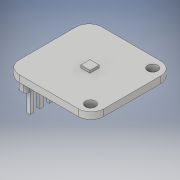
# Autodesk Inventor part: Adafruit TMP007 IR Sensor
Saved by Autodesk Inventor 2018 (Build 220112000, 112)
## iProperties
Created: 2018-10-23
Part Number: Adafruit TMP007 IR Sensor
Material: Generic
Document SubType Name: Modeling
Designer: tbrow
Density: 1 g/cm^3
Appearance: Default
Author: tbrow
Autodesk Inventor part; units mm, degrees
ref_plane "YZ Plane" through (0, 0, 0) normal (1, 0, 0) x (0, 1, 0)
ref_plane "XZ Plane" through (0, 0, 0) normal (0, 1, 0) x (-1, 0, 0)
ref_plane "XY Plane" through (0, 0, 0) normal (0, 0, 1) x (1, 0, 0)
sketch "Sketch1" plane through (0, 0, 0) normal (0, 1, 0) x (-1, 0, 0)
  line L0 (3.175, 0) -> (17.653, 0)
  line L1 (20.828, -3.175) -> (20.828, -17.145)
  line L2 (17.653, -20.32) -> (3.175, -20.32)
  line L3 (0, -17.145) -> (0, -3.175)
  circle A0 centre (2.6416, -2.5146) radius 1.2446
  circle A1 centre (2.6416, -17.8054) radius 1.2446
  line L4 (1.397, -2.5146) -> (0, -2.5146) construction
  line L5 (2.6416, -1.27) -> (2.6416, 0) construction
  line L6 (1.397, -17.8054) -> (0, -17.8054) construction
  line L7 (2.6416, -19.05) -> (2.6416, -20.32) construction
  arc A2 (0, -17.145) -> (3.175, -20.32) centre (3.175, -17.145) ccw
  arc A3 (3.175, 0) -> (0, -3.175) centre (3.175, -3.175) ccw
  arc A4 (20.828, -3.175) -> (17.653, 0) centre (17.653, -3.175) ccw
  arc A5 (17.653, -20.32) -> (20.828, -17.145) centre (17.653, -17.145) ccw
  point P0 (0, 0)
  point P1 (20.828, -20.32)
  point P2 (20.828, 0)
  point P3 (0, -20.32)
  dimension "d0" = 20.32
  dimension "d1" = 20.828
  dimension "d2" = 2.4892
  dimension "d3" = 2.4892
  dimension "d4" = 1.397
  dimension "d5" = 1.27
  dimension "d6" = 1.27
  dimension "d7" = 1.397
  dimension "d8" = 3.175
  constraints: 16 end point, 16 point on line, 12 point on circle, 8 tangent, 6 centre point, 4 perpendicular, 3 equal radius, 2 horizontal, 2 parallel
  measures "d0" distance of point (20.828, 0) point (20.828, -20.32)
  measures "d1" distance of point (20.828, -20.32) point (0, -20.32)
  measures "d2" diameter of A0
  measures "d3" diameter of A1
  measures "d4" distance of L4.start L4.end
  measures "d5" distance of L5.start L5.end
  measures "d6" distance of L7.start L7.end
  measures "d7" distance of L6.start L6.end
  measures "d8" radius of A2
extrude "Extrusion1" add sketch "Sketch1" along normal blind 1.651
sketch "Sketch2" plane through (0, 1.651, 0) normal (0, 1, 0) x (1, 0, 0)
  line L0 (-11.557, 9.017) -> (-9.271, 9.017)
  line L1 (-9.271, 9.017) -> (-9.271, 11.303)
  line L2 (-9.271, 11.303) -> (-11.557, 11.303)
  line L3 (-11.557, 11.303) -> (-11.557, 9.017)
  line L4 (-11.557, 10.16) -> (-9.271, 10.16) construction
  line L5 (-10.414, 9.017) -> (-10.414, 11.303) construction
  line L6 (-3.175, 20.32) -> (-17.653, 20.32) projected
  line L7 (-20.828, 17.145) -> (-20.828, 3.175) projected
  point P0 (0, 0)
  point P1 (-10.414, 20.32)
  point P2 (-20.828, 10.16)
  dimension "d11" = 2.286
  dimension "d12" = 2.286
  constraints: 12 end point, 6 midpoint, 2 parallel, 2 point on line, 1 horizontal, 1 perpendicular
  measures "d11" distance of L2.end L0.start
  measures "d12" distance of L1.end L2.end
extrude "Extrusion2" add sketch "Sketch2" along normal blind 0.5842
sketch "Sketch3" plane through (0, 0, 0) normal (0, -1, 0) x (1, 0, 0)
  line L0 (-18.3896, -19.431) -> (-17.6022, -19.431)
  line L1 (-16.8402, -18.669) -> (-16.8402, -1.651)
  line L2 (-17.6022, -0.889) -> (-18.3896, -0.889)
  line L3 (-19.1516, -1.651) -> (-19.1516, -18.669)
  line L4 (-17.653, -20.32) -> (-3.175, -20.32) projected
  line L5 (-3.175, 0) -> (-17.653, 0) projected
  line L6 (-20.828, -3.175) -> (-20.828, -17.145) projected
  arc A0 (-19.1516, -18.669) -> (-18.3896, -19.431) centre (-18.3896, -18.669) ccw
  arc A1 (-18.3896, -0.889) -> (-19.1516, -1.651) centre (-18.3896, -1.651) ccw
  arc A2 (-16.8402, -1.651) -> (-17.6022, -0.889) centre (-17.6022, -1.651) ccw
  arc A3 (-17.6022, -19.431) -> (-16.8402, -18.669) centre (-17.6022, -18.669) ccw
  point P0 (0, 0)
  dimension "d15" = 0.889
  dimension "d16" = 0.889
  dimension "d17" = 3.9878
  dimension "d18" = 1.6764
  dimension "d19" = 0.762
  constraints: 8 end point, 8 point on circle, 8 tangent, 4 centre point, 3 equal radius, 2 parallel, 1 horizontal, 1 perpendicular
  measures "d15" distance between parallel lines of L4 L0
  measures "d16" distance between parallel lines of L5 L2
  measures "d17" distance between parallel lines of L6 L1
  measures "d18" distance between parallel lines of L6 L3
  measures "d19" radius of A0
extrude "Extrusion3" add sketch "Sketch3" along normal blind 2.54
sketch "Sketch4" plane through (0, -2.54, 0) normal (0, -1, 0) x (1, 0, 0)
  line L0 (-18.415, -17.6657) -> (-17.5768, -17.6657)
  line L1 (-17.5768, -17.6657) -> (-17.5768, -16.8275)
  line L2 (-17.5768, -16.8275) -> (-18.415, -16.8275)
  line L3 (-18.415, -16.8275) -> (-18.415, -17.6657)
  line L4 (-17.9959, -17.6657) -> (-17.9959, -16.8275) construction
  line L5 (-18.3896, -19.431) -> (-17.6022, -19.431) projected
  line L6 (-18.415, -15.3035) -> (-17.5768, -15.3035)
  line L7 (-17.5768, -15.3035) -> (-17.5768, -14.4653)
  line L8 (-17.5768, -14.4653) -> (-18.415, -14.4653)
  line L9 (-18.415, -14.4653) -> (-18.415, -15.3035)
  line L10 (-17.9959, -15.3035) -> (-17.9959, -14.4653) construction
  line L11 (-18.415, -12.9413) -> (-17.5768, -12.9413)
  line L12 (-17.5768, -12.9413) -> (-17.5768, -12.1031)
  line L13 (-17.5768, -12.1031) -> (-18.415, -12.1031)
  line L14 (-18.415, -12.1031) -> (-18.415, -12.9413)
  line L15 (-17.9959, -12.9413) -> (-17.9959, -12.1031) construction
  line L16 (-18.415, -10.5791) -> (-17.5768, -10.5791)
  line L17 (-17.5768, -10.5791) -> (-17.5768, -9.7409)
  line L18 (-17.5768, -9.7409) -> (-18.415, -9.7409)
  line L19 (-18.415, -9.7409) -> (-18.415, -10.5791)
  line L20 (-17.9959, -10.5791) -> (-17.9959, -9.7409) construction
  line L21 (-18.415, -8.2169) -> (-17.5768, -8.2169)
  line L22 (-17.5768, -8.2169) -> (-17.5768, -7.3787)
  line L23 (-17.5768, -7.3787) -> (-18.415, -7.3787)
  line L24 (-18.415, -7.3787) -> (-18.415, -8.2169)
  line L25 (-17.9959, -8.2169) -> (-17.9959, -7.3787) construction
  line L26 (-18.415, -5.8547) -> (-17.5768, -5.8547)
  line L27 (-17.5768, -5.8547) -> (-17.5768, -5.0165)
  line L28 (-17.5768, -5.0165) -> (-18.415, -5.0165)
  line L29 (-18.415, -5.0165) -> (-18.415, -5.8547)
  line L30 (-17.9959, -5.8547) -> (-17.9959, -5.0165) construction
  line L31 (-18.415, -3.4925) -> (-17.5768, -3.4925)
  line L32 (-17.5768, -3.4925) -> (-17.5768, -2.6543)
  line L33 (-17.5768, -2.6543) -> (-18.415, -2.6543)
  line L34 (-18.415, -2.6543) -> (-18.415, -3.4925)
  line L35 (-17.9959, -3.4925) -> (-17.9959, -2.6543) construction
  line L36 (-18.415, -10.16) -> (-17.5768, -10.16) construction
  line L37 (-19.1516, -1.651) -> (-19.1516, -18.669) projected
  point P0 (0, 0)
  point P1 (-17.9959, -19.431)
  point P2 (-17.9959, -17.0688)
  point P3 (-17.9959, -14.7066)
  point P4 (-17.9959, -12.3444)
  point P5 (-17.9959, -9.9822)
  point P6 (-17.9959, -7.62)
  point P7 (-17.9959, -5.2578)
  point P8 (-19.1516, -10.16)
  dimension "d22" = 0.8382
  dimension "d23" = 0.8382
  dimension "d26" = 2.3622
  constraints: 72 end point, 8 point on line, 6 midpoint, 2 parallel, 1 collinear, 1 horizontal, 1 perpendicular, 1 vertical, 71 other
  measures "d22" distance of L2.end L0.start
  measures "d23" distance of L1.end L2.end
  measures "d26" distance of L0.start L6.start
extrude "Extrusion4" add sketch "Sketch4" along normal blind 5.842
chamfer "Chamfer1" distance 0.254 angle 45 28 edges at (-18.415, -8.382, -17.2466) (-17.9959, -8.382, -17.6657) (-17.5768, -8.382, -17.2466) (-17.9959, -8.382, -16.8275) (-18.415, -8.382, -14.8844) (-17.9959, -8.382, -15.3035) (-17.5768, -8.382, -14.8844) (-17.9959, -8.382, -14.4653) (-17.9959, -8.382, -12.9413) (-18.415, -8.382, -12.5222) (-17.9959, -8.382, -12.1031) (-17.5768, -8.382, -12.5222) (-17.5768, -8.382, -10.16) (-17.9959, -8.382, -9.7409) (-18.415, -8.382, -10.16) (-17.9959, -8.382, -10.5791) (-17.9959, -8.382, -8.2169) (-18.415, -8.382, -7.7978) (-17.9959, -8.382, -7.3787) (-17.5768, -8.382, -7.7978) (-18.415, -8.382, -5.4356) (-17.9959, -8.382, -5.0165) (-17.5768, -8.382, -5.4356) (-17.9959, -8.382, -5.8547) (-17.9959, -8.382, -3.4925) (-18.415, -8.382, -3.0734) (-17.9959, -8.382, -2.6543) (-17.5768, -8.382, -3.0734)
equation "\"d3\" = d2"
equation "\"d6\" = d5"
equation "\"d7\" = d4"
body "Solid1"
